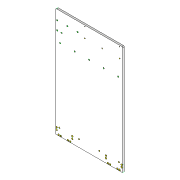
# Autodesk Inventor part: TL20240701-10120CV-002
Saved by Autodesk Inventor 2022.5 (Build 265521000, 521)
## iProperties
Category: FOLLOWER UNIT ASSY
Manager: 호상태
Company: 현대 트랜시스(대유)
RuleStatus: InUse
Created: 2023-01-19
Part Number: TL20240701-10120CV-002
Project: SW PJT
Checked By: 김형민
Engr Approved By: 김시현
User Status: 1/1 x18
Material: SS400
Description: 0
Document SubType Name: Modeling
Mfg Approved By: 호상태
Designer: 박성규
Stock Number: 002
Mass: 13148.3 g
Surface Area: 1560.92 cm^2
Volume: 1670.68 cm^3
Density: 7.85 g/cm^3
Appearance: Painting-RAL7035
BeforeDocSave0: file://Part Design STD iLogic
DETAIL: Coveryor Assembly
M/C TITLE: MEa/NEa차종 시트조립라인
SPECIFICATION: TL20221201-000000CV-005
DocNumber: 221118_Standard_v1
Folder: .\
VDS_Category: 엔지니어링
Detail Description: Processed products
Title: SIDE PLATE
Subject: SW차종 시트조립라인
Author: 박성규
Revision Number: A
Autodesk Inventor part; units mm, degrees
ref_plane "YZ Plane" through (0, 0, 0) normal (1, 0, 0) x (0, 1, 0)
ref_plane "XZ Plane" through (0, 0, 0) normal (0, 1, 0) x (-1, 0, 0)
ref_plane "XY Plane" through (0, 0, 0) normal (0, 0, 1) x (1, 0, 0)
sketch "스케치22" plane through (0, 0, 0) normal (0, 0, 1) x (1, 0, 0)
  line L0 (-230, 375) -> (230, 375)
  line L1 (230, 375) -> (230, -375)
  line L2 (230, -375) -> (-230, -375)
  line L3 (-230, -375) -> (-230, 375)
  line L4 (-230, 375) -> (230, -375) construction
  line L5 (230, 375) -> (-230, -375) construction
  point P0 (0, 0)
  dimension "d122" = 460
  dimension "HIGHT" = 750
  constraints: 12 end point, 2 midpoint, 2 parallel, 1 horizontal, 1 perpendicular
  measures "d122" distance of L0.start L0.end
  measures "HIGHT" distance of L0.end L1.end
extrude "돌출12" add sketch "스케치22" along normal blind 12
sketch "스케치23" plane through (0, 0, 12) normal (0, 0, 1) x (1, 0, 0)
  line L0 (230, 375) -> (-230, 375) construction
  line L1 (-230, 375) -> (-230, -375) construction
  point P0 (0, 0)
  point P1 (-220, 309)
  point P2 (-220, 249)
  point P3 (-190, 249)
  point P4 (-150, 309)
  point P5 (-80, 309)
  point P6 (-220, -261)
  point P7 (-150, -261)
  point P8 (-80, -261)
  point P9 (-220, -321)
  point P10 (-190, -321)
  dimension "d126" = 66
  dimension "d128" = 126
  dimension "d129" = 10
  dimension "d130" = 10
  dimension "d131" = 70
  dimension "d132" = 70
  dimension "d133" = 30
  dimension "d154" = 10
  dimension "d155" = 30
  dimension "d156" = 696
  dimension "d157" = 636
  dimension "d158" = 10
  dimension "d159" = 70
  dimension "d160" = 70
  constraints: 6 horizontal alignment
  measures "d126" distance from line of L0 point (-220, 309)
  measures "d128" distance from line of L0 point (-220, 249)
  measures "d129" distance from line of L1 point (-220, 309)
  measures "d130" distance from line of L1 point (-220, 249)
  measures "d131" distance of point (-150, 309) point (-220, 309)
  measures "d132" distance of point (-80, 309) point (-150, 309)
  measures "d133" distance of point (-190, 249) point (-220, 249)
  measures "d154" distance from line of L1 point (-220, -321)
  measures "d155" distance of point (-220, -321) point (-190, -321)
  measures "d156" distance from line of L0 point (-220, -321)
  measures "d157" distance from line of L0 point (-220, -261)
  measures "d158" distance from line of L1 point (-220, -261)
  measures "d159" distance of point (-150, -261) point (-220, -261)
  measures "d160" distance of point (-80, -261) point (-150, -261)
hole "구멍7" at (-220, 309, 12) at (-220, 249, 12) at (-190, 249, 12) at (-150, 309, 12) at (-80, 309, 12) direction (0, 0, -1) diameter 9 end through all clearance for "Socket Head Cap Screw" size "M8" standard "TS Profile"
sketch "스케치24" plane through (0, 0, 12) normal (0, 0, 1) x (1, 0, 0)
  line L0 (230, 375) -> (-230, 375) construction
  line L1 (-230, 375) -> (-230, -375) construction
  line L2 (230, -375) -> (230, 375) construction
  line L3 (-230, -375) -> (230, -375) projected
  point P0 (0, 0)
  point P1 (-200, 183)
  point P2 (-100, 183)
  point P3 (0, 183)
  point P4 (100, 183)
  point P5 (200, 183)
  point P6 (55, -357)
  point P7 (0, -357)
  point P8 (-55, -357)
  point P9 (-110, -357)
  point P10 (110, -357)
  dimension "d141" = 30
  dimension "d142" = 192
  dimension "d143" = 100
  dimension "d144" = 100
  dimension "d145" = 100
  dimension "d146" = 100
  dimension "d231" = 55
  dimension "d234" = 120
  dimension "d308" = 120
  dimension "d338" = 18
  dimension "d339" = 55
  dimension "d340" = 55
  dimension "d341" = 55
  constraints: 8 horizontal alignment
  measures "d141" distance from line of L1 point (-200, 183)
  measures "d142" distance from line of L0 point (-200, 183)
  measures "d143" distance of point (-100, 183) point (-200, 183)
  measures "d144" distance of point (0, 183) point (-100, 183)
  measures "d145" distance of point (0, 183) point (100, 183)
  measures "d146" distance of point (200, 183) point (100, 183)
  measures "d231" distance of point (-55, -357) point (-110, -357)
  measures "d234" distance from line of L1 point (-110, -357)
  measures "d308" distance from line of L2 point (110, -357)
  measures "d338" distance from line of point (-110, -357) L3
  measures "d339" distance of point (0, -357) point (55, -357)
  measures "d340" distance of point (-55, -357) point (0, -357)
  measures "d341" distance of point (55, -357) point (110, -357)
hole "구멍8" at (-200, 183, 12) at (-100, 183, 12) at (0, 183, 12) at (100, 183, 12) at (200, 183, 12) direction (0, 0, -1) diameter 9 end through all clearance for "Socket Head Cap Screw" size "M8" standard "TS Profile"
fillet "모깎기6" radius 5 2 edges at (-230, 375, 6) (230, 375, 6)
sketch "스케치29" plane through (0, 0, 12) normal (0, 0, 1) x (1, 0, 0)
  line L0 (230, -375) -> (230, 370) construction
  line L1 (225, 375) -> (-225, 375) construction
  point P0 (0, 0)
  point P1 (210, 367)
  point P2 (-30, 367)
  point P3 (210, -203)
  point P4 (-30, -203)
  dimension "d199" = 8
  dimension "d200" = 20
  dimension "d201" = 240
  dimension "d202" = 570
  constraints: 2 horizontal alignment, 2 vertical alignment
  measures "d199" distance from line of L1 point (210, 367)
  measures "d200" distance from line of L0 point (210, 367)
  measures "d201" distance of point (-30, 367) point (210, 367)
  measures "d202" distance of point (210, -203) point (210, 367)
hole "구멍11" at (210, 367, 12) at (-30, 367, 12) direction (0, 0, -1) diameter 4.917 end through all thread size "M6x1" class "6H" standard "TS profile"
sketch "스케치31" plane through (0, 0, 0) normal (0, 0, -1) x (-1, 0, 0)
  line L0 (-230, -375) -> (-230, 370) construction
  line L1 (-225, 375) -> (225, 375) construction
  point P0 (-75, 375)
  point P1 (-162, 375)
  point P2 (0, 0)
  point P3 (-210, 296)
  point P4 (-90, 296)
  point P5 (30, 296)
  point P6 (-198, 375)
  point P7 (-196, 375)
  dimension "d219" = 79
  dimension "d220" = 20
  dimension "d221" = 120
  dimension "d222" = 120
  constraints: 2 horizontal alignment
  measures "d219" distance from line of point (-210, 296) L1
  measures "d220" distance from line of L0 point (-210, 296)
  measures "d221" distance of point (-90, 296) point (-210, 296)
  measures "d222" distance of point (-90, 296) point (30, 296)
hole "구멍13" at (210, 296, 0) at (90, 296, 0) at (-30, 296, 0) direction (0, 0, 1) diameter 6.6 end through all clearance for "Socket Head Cap Screw" size "M6" standard "TS Profile"
sketch "스케치43" plane through (0, 0, 0) normal (0, 0, -1) x (-1, 0, 0)
  line L0 (230, 370) -> (230, -375) projected
  line L1 (230, -375) -> (-230, -375) projected
  point P0 (0, 0)
  point P1 (205, -325)
  point P2 (70, -325)
  point P3 (-70, -325)
  point P4 (-205, -325)
  dimension "d309" = 135
  dimension "d310" = 140
  dimension "d311" = 135
  dimension "d312" = 25
  dimension "d314" = 50
  constraints: 3 horizontal alignment
  measures "d309" distance of point (70, -325) point (205, -325)
  measures "d310" distance of point (-70, -325) point (70, -325)
  measures "d311" distance of point (-205, -325) point (-70, -325)
  measures "d312" distance from line of L0 point (205, -325)
  measures "d314" distance from line of L1 point (205, -325)
hole "구멍18" at (-205, -325, 0) at (-70, -325, 0) at (70, -325, 0) at (205, -325, 0) direction (0, 0, 1) diameter 9 end through all clearance for "Socket Head Cap Screw" size "M8" standard "TS Profile"
sketch "스케치44" plane through (0, 0, 12) normal (0, 0, 1) x (1, 0, 0)
  line L0 (-116, -346) -> (-224, -346)
  line L1 (-224, -346) -> (-224, -331)
  line L2 (-224, -331) -> (-116, -331)
  line L3 (-116, -331) -> (-116, -346)
  line L4 (-116, -346) -> (-224, -331) construction
  line L5 (-224, -346) -> (-116, -331) construction
  line L6 (-230, 370) -> (-230, -375) projected
  line L7 (-230, -375) -> (230, -375) projected
  point P0 (0, 0)
  point P1 (-210, -369)
  point P2 (-195, -369)
  point P3 (-145, -369)
  point P4 (-130, -369)
  point P5 (-170, -338.5)
  dimension "d322" = 108
  dimension "d323" = 15
  dimension "d324" = 20
  dimension "d325" = 15
  dimension "d326" = 50
  dimension "d327" = 15
  dimension "d328" = 6
  dimension "d329" = 29
  dimension "d330" = 6
  constraints: 12 end point, 3 horizontal alignment, 2 midpoint, 2 parallel, 1 horizontal, 1 perpendicular
  measures "d322" distance of L0.start L0.end
  measures "d323" distance of L2.end L0.start
  measures "d324" distance from line of L6 point (-210, -369)
  measures "d325" distance of point (-195, -369) point (-210, -369)
  measures "d326" distance of point (-145, -369) point (-195, -369)
  measures "d327" distance of point (-130, -369) point (-145, -369)
  measures "d328" distance between parallel lines of L6 L1
  measures "d329" distance between parallel lines of L7 L0
  measures "d330" distance from line of L7 point (-210, -369)
hole "구멍19" at (-210, -369, 12) at (-195, -369, 12) at (-145, -369, 12) at (-130, -369, 12) at (-224, -346, 12) at (-224, -331, 12) at (-116, -346, 12) at (-116, -331, 12) direction (0, 0, -1) diameter 6.6 end through all counterbore diameter 11 counterbore depth 6.5 clearance for "Socket Head Cap Screw" size "M6" standard "TS Profile"
mirror "미러2" about plane through (0, 0, 0) normal (1, 0, 0) of "구멍19"
equation "\"d132\" = d131"
equation "\"d160\" = d159"
equation "\"d144\" = d143"
equation "\"d145\" = d143"
equation "\"d146\" = d143"
